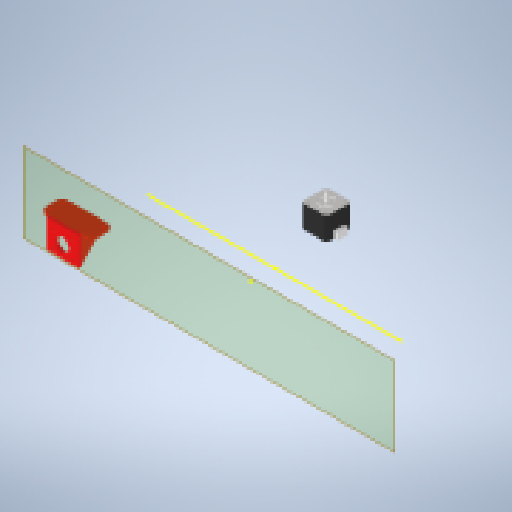
# Autodesk Inventor part: steppeSquare
Saved by Autodesk Inventor 2023 (Build 270158000, 158)
## iProperties
Created: 2020-10-13
Part Number: steppeSquare
Material: Generic
Document SubType Name: Modeling
Designer: Felix
Density: 1 g/cm^3
Appearance: Default
Author: Felix
Autodesk Inventor part; units mm, degrees
ref_plane "YZ Plane" through (0, 0, 0) normal (1, 0, 0) x (0, 1, 0)
ref_plane "XZ Plane" through (0, 0, 0) normal (0, 1, 0) x (-1, 0, 0)
ref_plane "XY Plane" through (0, 0, 0) normal (0, 0, 1) x (1, 0, 0)
sketch "Sketch1" plane through (0, 0, 0) normal (0, 1, 0) x (-1, 0, 0)
  line L0 (21, 21) -> (-21, 21)
  line L1 (-21, 21) -> (-21, -21)
  line L2 (-21, -21) -> (21, -21)
  line L3 (21, -21) -> (21, 21)
  line L4 (21, 21) -> (-21, -21) construction
  line L5 (-21, 21) -> (21, -21) construction
  point P0 (0, 0)
  dimension "d0" = 42
  dimension "d1" = 42
  constraints: 12 end point, 2 midpoint, 2 parallel, 1 horizontal, 1 perpendicular
  measures "d0" distance of L2.end L1.end
  measures "d1" distance of L1.end L0.end
extrude "Extrusion1" add sketch "Sketch1" along normal blind 37.5
fillet "Fillet1" radius 5 4 edges at (21, 18.75, 21) (21, 18.75, -21) (-21, 18.75, -21) (-21, 18.75, 21)
sketch "Sketch2" plane through (0, 37.5, 0) normal (0, 1, 0) x (1, 0, 0)
  arc A0 (-21, -16) -> (-16, -21) centre (-16, -16) ccw projected
  line L0 (-16, -21) -> (16, -21) projected
  arc A1 (16, -21) -> (21, -16) centre (16, -16) ccw projected
  line L1 (21, -16) -> (21, 16) projected
  arc A2 (21, 16) -> (16, 21) centre (16, 16) ccw projected
  line L2 (16, 21) -> (-16, 21) projected
  arc A3 (-16, 21) -> (-21, 16) centre (-16, 16) ccw projected
  line L3 (-21, 16) -> (-21, -16) projected
  circle A4 centre (0, 0) radius 11
  circle A5 centre (0, 0) radius 10
  point P0 (-15, -15)
  point P1 (15, -15)
  point P2 (15, 15)
  point P3 (-15, 15)
  dimension "d5" = 22
  dimension "d6" = 20
  dimension "d7" = 6
  dimension "d8" = 6
  dimension "d11" = 360
  constraints: 2 centre point, 2 coincident, 5 other
  measures "d5" diameter of A4
  measures "d6" diameter of A5
  measures "d7" distance from line of point (-15, -15) L0
  measures "d8" distance from line of L3 point (-15, -15)
extrude "Extrusion2" add sketch "Sketch2" along normal blind 2 contours A4
hole "Hole1" at (-15, 37.5, 15) at (15, 37.5, 15) at (15, 37.5, -15) at (-15, 37.5, -15) direction (0, -1, 0) diameter 2.459 depth 8.8 thread size "M3x0.5" class "6H" standard "ISO Metric profile"
sketch "Sketch3" plane through (0, 37.5, 0) normal (0, 1, 0) x (1, 0, 0)
  circle A0 centre (0, 0) radius 2.5
  dimension "d22" = 5
  constraints: 1 centre point, 1 coincident
  measures "d22" diameter of A0
extrude "Extrusion3" add sketch "Sketch3" along normal blind 6
chamfer "Chamfer1" distance 0.5 angle 45 1 edges at (-2.5, 43.5, 0)
sketch "Sketch4" plane through (0, 43.5, 0) normal (0, 1, 0) x (1, 0, 0)
  line L0 (-1.5, 1.5) -> (1.5, 1.5)
  line L1 (1.5, 1.5) -> (1.5, -1.5)
  line L2 (1.5, -1.5) -> (-1.5, -1.5)
  line L3 (-1.5, -1.5) -> (-1.5, 1.5)
  line L4 (-1.5, 1.5) -> (1.5, -1.5) construction
  line L5 (1.5, 1.5) -> (-1.5, -1.5) construction
  point P0 (0, 0)
  dimension "d28" = 3
  dimension "d29" = 3
  constraints: 12 end point, 2 midpoint, 2 parallel, 1 horizontal, 1 perpendicular
  measures "d28" distance of L1.end L2.end
  measures "d29" distance of L0.end L1.end
extrude "Extrusion4" add sketch "Sketch4" along normal blind 8.6
sketch "Sketch5" plane through (21, 0, 16) normal (1, 0, 0) x (0, 0, -1)
  line L0 (7.5, 12) -> (24.5, 12)
  line L1 (24.5, 12) -> (24.5, 0)
  line L2 (24.5, 0) -> (7.5, 0)
  line L3 (7.5, 0) -> (7.5, 12)
  line L4 (7.5, 12) -> (24.5, 0) construction
  line L5 (24.5, 12) -> (7.5, 0) construction
  line L6 (0, 0) -> (32, 0) projected
  point P0 (16, 0)
  point P1 (16, 6)
  point P2 (16, 0)
  dimension "d32" = 17
  dimension "d33" = 12
  constraints: 12 end point, 4 midpoint, 2 parallel, 1 horizontal, 1 perpendicular
  measures "d32" distance between parallel lines of L1 L3
  measures "d33" distance of L0.end L1.end
extrude "Extrusion5" add sketch "Sketch5" along normal blind 6
body "Solid1"
